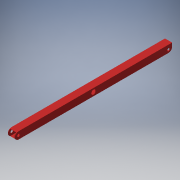
# Autodesk Inventor part: Front lift arm
Saved by Autodesk Inventor 2017 SP1 (Build 210196100, 196)
## iProperties
Created: 2018-01-12
Part Number: Front lift arm
Material: Aluminum 6061
Document SubType Name: Modeling
Designer: Ben
Density: 2.7 g/cm^3
Appearance: Light Red
Author: Ben
Autodesk Inventor part; units mm, degrees
ref_plane "YZ Plane" through (0, 0, 0) normal (1, 0, 0) x (0, 1, 0)
ref_plane "XZ Plane" through (0, 0, 0) normal (0, 1, 0) x (-1, 0, 0)
ref_plane "XY Plane" through (0, 0, 0) normal (0, 0, 1) x (1, 0, 0)
sketch "Sketch1" plane through (0, 0, 0) normal (0, 0, 1) x (1, 0, 0)
  line L0 (-12.7, -12.7) -> (12.7, -12.7)
  line L1 (12.7, -12.7) -> (12.7, 12.7)
  line L2 (12.7, 12.7) -> (-12.7, 12.7)
  line L3 (-12.7, 12.7) -> (-12.7, -12.7)
  line L4 (-12.7, -12.7) -> (12.7, 12.7) construction
  line L5 (12.7, -12.7) -> (-12.7, 12.7) construction
  line L6 (-11.1125, -11.1125) -> (11.1125, -11.1125)
  line L7 (11.1125, -11.1125) -> (11.1125, 11.1125)
  line L8 (11.1125, 11.1125) -> (-11.1125, 11.1125)
  line L9 (-11.1125, 11.1125) -> (-11.1125, -11.1125)
  line L10 (-11.1125, -11.1125) -> (11.1125, 11.1125) construction
  line L11 (11.1125, -11.1125) -> (-11.1125, 11.1125) construction
  point P0 (0, 0)
  dimension "d0" = 25.4
  dimension "d1" = 25.4
  dimension "d2" = 1.5875
  constraints: 24 end point, 4 midpoint, 4 parallel, 2 horizontal, 2 perpendicular, 1 collinear
  measures "d0" distance of L0.start L0.end
  measures "d1" distance of L0.end L1.end
  measures "d2" distance between parallel lines of L1 L7
extrude "Extrusion1" add sketch "Sketch1" along normal mid plane 558.8
sketch "Sketch2" plane through (-12.7, -12.7, 279.4) normal (-1, 0, 0) x (0, 0, 1)
  circle A0 centre (-279.4, 12.7) radius 7.9375
  line L0 (-558.8, 12.7) -> (0, 12.7) construction
  line L1 (0, 1.5875) -> (0, 23.8125) construction
  circle A1 centre (-546.1, 9.8186) radius 4.7625
  line L2 (-546.1, 0) -> (-558.8, 0)
  arc A2 (-558.8, 12.7) -> (-546.1, 0) centre (-546.1, 12.7) ccw
  line L3 (-558.8, 12.7) -> (-558.8, 0)
  line L4 (-558.8, 25.4) -> (0, 25.4) construction
  line L5 (-279.4, 25.4) -> (-279.4, 0) construction
  circle A3 centre (-12.7, 12.7) radius 4.7625
  arc A4 (-12.7, 0) -> (0, 12.7) centre (-12.7, 12.7) ccw
  arc A5 (0, 12.7) -> (-12.7, 25.4) centre (-12.7, 12.7) ccw
  line L6 (-12.7, 25.4) -> (0, 25.4)
  line L7 (0, 25.4) -> (0, 12.7)
  line L8 (0, 12.7) -> (0, 0)
  line L9 (0, 0) -> (-12.7, 0)
  line L10 (-558.8, 0) -> (-558.8, 25.4) construction
  line L11 (0, 0) -> (-558.8, 0) construction
  circle A6 centre (-546.1, 9.8186) radius 12.7 construction
  dimension "d5" = 15.875
  dimension "d6" = 9.525
  dimension "d13" = 12.7
  dimension "d14" = 9.8186
  dimension "d15" = 25.4
  constraints: 16 end point, 7 centre point, 6 point on circle, 5 tangent, 4 point on line, 3 coincident, 3 midpoint, 2 collinear, 2 horizontal, 2 perpendicular, 1 equal radius, 1 vertical
  measures "d5" diameter of A0
  measures "d6" diameter of A1
  measures "d13" distance from line of L10 A1.centre
  measures "d14" distance from line of L11 A1.centre
  measures "d15" diameter of A6
extrude "Extrusion2" cut sketch "Sketch2" against normal through all
sketch "Sketch4" plane through (0, 0, 0) normal (0, 1, 0) x (-1, 0, 0)
  line L0 (-12.7, -266.7) -> (12.7, -266.7) construction
  line L1 (11.1125, -290.9216) -> (-11.1125, -290.9216)
  line L2 (-11.1125, -290.9216) -> (-11.1125, -254)
  line L3 (-11.1125, -254) -> (11.1125, -254)
  line L4 (11.1125, -254) -> (11.1125, -290.9216)
  line L5 (-11.1125, 272.8484) -> (11.1125, 272.8484) construction
  line L6 (11.1125, -279.4) -> (11.1125, 272.8484) construction
  line L7 (-11.1125, -279.4) -> (11.1125, -279.4) construction
  line L8 (-11.1125, -279.4) -> (-11.1125, 272.8484) construction
  point P0 (0, 0)
  dimension "d16" = 12.7
  constraints: 8 end point, 2 collinear, 2 parallel, 1 horizontal, 1 perpendicular
  measures "d16" distance between parallel lines of L0 L3
extrude "Extrusion4" cut sketch "Sketch4" against normal through all
body "Solid1"
